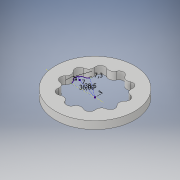
# Autodesk Inventor part: Enclosure
Saved by Autodesk Inventor 2018.3 (Build 223284000, 284)
## iProperties
Created: 2018-07-20
Part Number: Enclosure
Material: Generisch
Document SubType Name: Modeling
Designer: JochenAlt
Density: 1 g/cm^3
Appearance: Vorgabe
Author: JochenAlt
Autodesk Inventor part; units mm, degrees
ref_plane "YZ Plane" through (0, 0, 0) normal (1, 0, 0) x (0, 1, 0)
ref_plane "XZ Plane" through (0, 0, 0) normal (0, 1, 0) x (-1, 0, 0)
ref_plane "XY Plane" through (0, 0, 0) normal (0, 0, 1) x (1, 0, 0)
sketch "Skizze1" plane through (0, 0, 0) normal (0, 0, 1) x (1, 0, 0)
  line L0 (-64.7124, 0) -> (10.7854, 0) construction
  arc A0 (-41.6874, 30.2877) -> (-51.5284, 0) centre (0, 0) ccw
  arc A1 (-31.5, 0) -> (-33.7731, 5.163) centre (-38.5, 0) ccw
  line L1 (0, 0) -> (-36.5327, 26.5426) construction
  line L2 (-38.5, 0) -> (0, 0) construction
  arc A2 (-30.3577, 15.6744) -> (-25.484, 18.5152) centre (-31.1472, 22.6297) ccw
  arc A3 (-37.8636, 6.971) -> (-38.5, 0) centre (0, 0) ccw construction
  arc A4 (-31.1472, 22.6297) -> (-37.8636, 6.971) centre (0, 0) ccw construction
  line L3 (-37.3909, 12.1491) -> (0, 0) construction
  arc A5 (-30.3577, 15.6744) -> (-33.7731, 5.163) centre (-29.673, 9.6413) ccw
  line L4 (-25.484, 18.5152) -> (-41.6874, 30.2877)
  line L5 (-31.5, 0) -> (-51.5284, 0)
  point P0 (-36.6157, 11.8972)
  dimension "d5" = 7
  dimension "d14" = 38.5
  dimension "d28" = 36
  dimension "d36" = 7.3
  constraints: 15 point on circle, 10 end point, 6 centre point, 6 point on line, 2 coincident, 1 collinear, 1 equal radius, 1 tangent, 1 other
  measures "d5" radius of A1
  measures "d14" distance of L1.start L2.start
  measures "d28" angle of L1 L0
  measures "d36" distance of point (-36.616, 11.897) A5.centre
extrude "Extrusion1" add sketch "Skizze1" along normal blind 10
pattern_circular "Runde Anordnung1" count 10 over 360 about axis through (0, 0, 0) along (0, 0, 1) of "Extrusion1"
